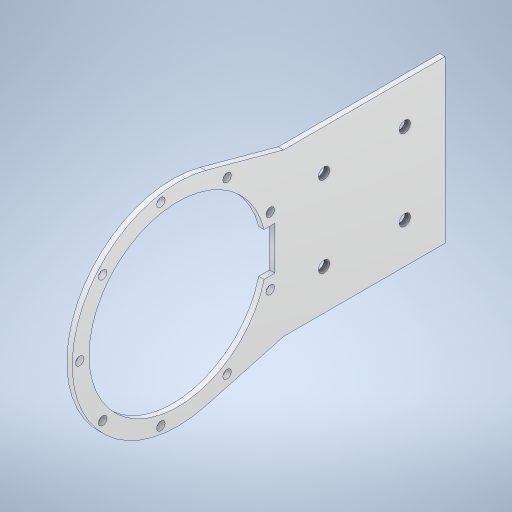
# Autodesk Inventor part: link3_plate2
Saved by Autodesk Inventor 2024 (Build 280153000, 153)
## iProperties
Created: 2024-12-13
Part Number: link3_plate2
Material: アルミニウム 6061
Document SubType Name: Modeling
Designer: hirek
Density: 2.7 g/cm^3
Appearance: アルミニウム - フラット
Author: hirek
Autodesk Inventor part; units mm, degrees
ref_plane "YZ Plane" through (0, 0, 0) normal (1, 0, 0) x (0, 1, 0)
ref_plane "XZ Plane" through (0, 0, 0) normal (0, 1, 0) x (-1, 0, 0)
ref_plane "XY Plane" through (0, 0, 0) normal (0, 0, 1) x (1, 0, 0)
sketch "スケッチ1" plane through (0, 0, 0) normal (1, 0, 0) x (0, 1, 0)
  circle A0 centre (0, 0) radius 39.25
  circle A1 centre (0, 0) radius 33
  line L0 (8, 0) -> (-8, 0)
  line L1 (-8, 0) -> (-8, -36)
  line L2 (-8, -36) -> (8, -36)
  line L3 (8, -36) -> (8, 0)
  line L4 (30, -39.25) -> (-30, -39.25)
  line L5 (-30, -39.25) -> (-30, -99.25)
  line L6 (-30, -99.25) -> (30, -99.25)
  line L7 (30, -99.25) -> (30, -39.25)
  line L8 (30, -39.25) -> (37.874, -10.3018)
  line L9 (-30, -39.25) -> (-37.874, -10.3018)
  point P0 (8, 32.0156)
  point P1 (8, -32.0156)
  point P2 (-8, -32.0156)
  point P3 (-8, 32.0156)
  point P4 (0, -39.25)
  dimension "d0" = 78.5
  dimension "d1" = 66
  dimension "d2" = 16
  dimension "d3" = 36
  dimension "d4" = 8
  dimension "d5" = 0
  dimension "d6" = 60
  dimension "d7" = 60
  dimension "d8" = 30
  dimension "d9" = 39.25
  constraints: 20 end point, 4 parallel, 2 centre point, 2 coincident, 2 horizontal, 2 perpendicular, 2 point on circle, 2 tangent
  measures "d0" diameter of A0
  measures "d1" diameter of A1
  measures "d2" distance of L2.end L1.end
  measures "d3" distance of L1.end L0.end
  measures "d4" distance from line of point (0, 0) L3
  measures "d5" distance from line of point (0, 0) L0
  measures "d6" distance of L6.end L5.end
  measures "d7" distance of L5.end L4.end
  measures "d8" distance from line of L7 point (0, 0)
  measures "d9" distance from line of L4 point (0, 0)
extrude "押し出し1" add sketch "スケッチ1" along normal blind 2
sketch "スケッチ2" plane through (2, 0, 0) normal (1, 0, 0) x (0, 0, -1)
  circle A0 centre (0, 0) radius 36.5
  point P0 (-36.5, 0)
  point P1 (-27.9606, -23.4617)
  point P2 (-6.3382, -35.9455)
  point P3 (18.25, -31.6099)
  point P4 (34.2988, -12.4837)
  point P5 (34.2988, 12.4837)
  point P6 (18.25, 31.6099)
  point P7 (-6.3382, 35.9455)
  point P8 (-27.9606, 23.4617)
  dimension "d12" = 73
  dimension "d15" = 360
  constraints: 1 coincident, 1 horizontal alignment, 12 other
hole "穴1" at (2, 0, 36.5) at (2, -23.4617, 27.9606) at (2, -35.9455, 6.3382) at (2, -31.6099, -18.25) at (2, -12.4837, -34.2988) at (2, 12.4837, -34.2988) at (2, 31.6099, -18.25) at (2, 35.9455, 6.3382) at (2, 23.4617, 27.9606) direction (-1, 0, 0) diameter 3.2 end through all
sketch "スケッチ3" plane through (2, 0, 0) normal (1, 0, 0) x (0, 0, -1)
  line L0 (54.25, 15) -> (84.25, 15)
  line L1 (84.25, 15) -> (84.25, -15)
  line L2 (84.25, -15) -> (54.25, -15)
  line L3 (54.25, -15) -> (54.25, 15)
  line L4 (99.25, -30) -> (99.25, 30) projected
  point P0 (0, 0)
  dimension "d24" = 30
  dimension "d25" = 30
  dimension "d26" = 15
  dimension "d27" = 15
  constraints: 8 end point, 4 coincident, 2 parallel, 1 horizontal, 1 perpendicular
  measures "d24" distance of L1.end L2.end
  measures "d25" distance of L0.end L1.end
  measures "d26" distance from line of L0 point (0, 0)
  measures "d27" distance between parallel lines of L1 L4
hole "穴2" at (2, 15, -54.25) at (2, -15, -54.25) at (2, 15, -84.25) at (2, -15, -84.25) direction (-1, 0, 0) diameter 4.2 end through all
